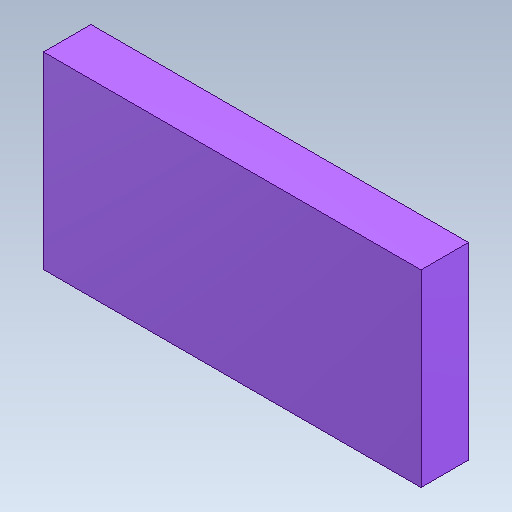
# Autodesk Inventor part: 0_22
Saved by Autodesk Inventor 2020 (Build 240168000, 168)
## iProperties
Created: 2019-08-29
Part Number: 0_22
Material: Generic
Document SubType Name: Modeling
Designer: psrob
Density: 1 g/cm^3
Appearance: R2512, 0_22
Author: psrob
Autodesk Inventor part; units mm, degrees
ref_plane "YZ Plane" through (0, 0, 0) normal (1, 0, 0) x (0, 1, 0)
ref_plane "XZ Plane" through (0, 0, 0) normal (0, 1, 0) x (-1, 0, 0)
ref_plane "XY Plane" through (0, 0, 0) normal (0, 0, 1) x (1, 0, 0)
sketch "R2512, 0_22_34" plane through (0, 0, 0) normal (0, 0, 1) x (1, 0, 0)
  line L0 (-3.973, 1.983) -> (3.973, 1.983)
  line L1 (3.973, 1.983) -> (3.973, -1.983)
  line L2 (3.973, -1.983) -> (-3.973, -1.983)
  line L3 (-3.973, -1.983) -> (-3.973, 1.983)
  constraints: 8 end point
extrude "Extrusion1" add sketch "R2512, 0_22_34" along normal blind 1
body "Solid1"
